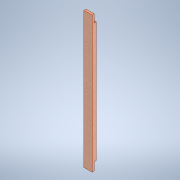
# Autodesk Inventor part: door side
Saved by Autodesk Inventor 2020 (Build 240168000, 168)
## iProperties
Created: 2020-05-09
Part Number: door side
Material: Wood (Oak)
Document SubType Name: Modeling
Designer: kolbe
Density: 0.76 g/cm^3
Appearance: White Oak - Natural Medium Gloss
Author: kolbe
Autodesk Inventor part; units mm, degrees
ref_plane "YZ Plane" through (0, 0, 0) normal (1, 0, 0) x (0, 1, 0)
ref_plane "XZ Plane" through (0, 0, 0) normal (0, 1, 0) x (-1, 0, 0)
ref_plane "XY Plane" through (0, 0, 0) normal (0, 0, 1) x (1, 0, 0)
sketch "Sketch1" plane through (0, 0, 0) normal (1, 0, 0) x (0, 1, 0)
  line L0 (0, 0) -> (863.6, 0)
  line L1 (863.6, 0) -> (863.6, -12.7)
  line L2 (863.6, -12.7) -> (812.8, -12.7)
  line L3 (812.8, -12.7) -> (812.8, -25.4)
  line L4 (812.8, -25.4) -> (50.8, -25.4)
  line L5 (50.8, -25.4) -> (50.8, -12.7)
  line L6 (50.8, -12.7) -> (0, -12.7)
  line L7 (0, -12.7) -> (0, 0)
  dimension "d0" = 863.6
  dimension "d1" = 12.7
  dimension "d2" = 50.8
  dimension "d3" = 12.7
  dimension "d4" = 762
  dimension "d5" = 12.7
  constraints: 16 end point, 5 perpendicular, 2 horizontal, 1 point on line
  measures "d0" distance of L0.start L0.end
  measures "d1" distance of L0.end L1.end
  measures "d2" distance of L1.end L2.end
  measures "d3" distance of L2.end L3.end
  measures "d4" distance of L3.end L4.end
  measures "d5" distance of L4.end L5.end
extrude "Extrusion1" add sketch "Sketch1" along normal blind 50.8
body "Solid1"
